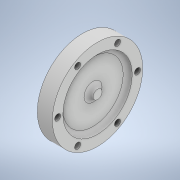
# Autodesk Inventor part: 711126 (Доделать)
Saved by Autodesk Inventor 2022 (Build 260153000, 153)
## iProperties
Created: 2021-10-21
Part Number: 711126 (Доделать)
Material: Типовые
Document SubType Name: Modeling
Designer: RaNSiD
Density: 1 g/cm^3
Appearance: По умолчанию
Author: RaNSiD
Autodesk Inventor part; units mm, degrees
ref_plane "YZ Plane" through (0, 0, 0) normal (1, 0, 0) x (0, 1, 0)
ref_plane "XZ Plane" through (0, 0, 0) normal (0, 1, 0) x (-1, 0, 0)
ref_plane "XY Plane" through (0, 0, 0) normal (0, 0, 1) x (1, 0, 0)
sketch "Эскиз1" plane through (0, 0, 0) normal (0, 0, 1) x (1, 0, 0)
  line L0 (0, 0) -> (10, 0)
  line L1 (10, 0) -> (10, 30)
  line L2 (10, 30) -> (0, 30)
  line L3 (0, 30) -> (0, 0)
  dimension "d0" = 10
  dimension "d1" = 30
  constraints: 8 end point, 2 parallel, 1 horizontal, 1 perpendicular
  measures "d0" distance of L2.end L1.end
  measures "d1" distance of L1.end L0.end
revolve "Вращение1" add sketch "Эскиз1" angle 360 about axis through (0, 0, 0) along (1, 0, 0)
sketch "Эскиз2" plane through (0, 0, 0) normal (0, 0, 1) x (1, 0, 0)
  line L0 (0, 0) -> (10, 0)
  line L1 (10, -30) -> (10, 30) projected
  arc A0 (3, 20) -> (0, 23) centre (0, 20) ccw
  line L2 (3, 20) -> (0, 20) construction
  line L3 (0, 23) -> (0, 20) construction
  line L4 (7, 20) -> (7, 10)
  arc A1 (7, 6) -> (10, 3) centre (10, 6) ccw
  line L5 (7, 6) -> (10, 6) construction
  line L6 (10, 3) -> (10, 6) construction
  arc A2 (10, 23) -> (7, 20) centre (10, 20) ccw
  line L7 (7, 20) -> (10, 20) construction
  line L8 (10, 23) -> (10, 20) construction
  line L9 (7, 10) -> (7, 6)
  line L10 (0, -30) -> (0, 30) projected
  line L11 (0, 0) -> (0, 23)
  line L12 (10, 3) -> (10, 23)
  line L13 (3, 20) -> (3, 0)
  point P0 (10, 3)
  point P1 (10, 23)
  dimension "d4" = 3
  dimension "d5" = 90
  dimension "d6" = 3
  dimension "d7" = 90
  dimension "d8" = 3
  dimension "d9" = 90
  dimension "d10" = 3
  dimension "d12" = 20
  dimension "d14" = 20
  constraints: 24 end point, 6 point on circle, 5 tangent, 3 centre point, 2 vertical, 2 vertical alignment, 1 horizontal alignment, 1 midpoint, 1 perpendicular, 1 point on line
  measures "d4" radius of A0
  measures "d5" angle of L2 L3
  measures "d6" radius of A1
  measures "d7" angle of L5 L6
  measures "d8" radius of A2
  measures "d9" angle of L8 L7
  measures "d10" distance of L0.end L6.start
  measures "d12" diameter of L4.end L0
  measures "d14" distance of L2.start L13.end
revolve "Вращение2" cut sketch "Эскиз2" angle 360 about axis through (0, 0, 0) along (-1, 0, 0) contours A1 L9 L4 A2 L1
sketch "Эскиз3" plane through (10, 0, 0) normal (1, 0, 0) x (0, 0, -1)
  point P0 (0, 0)
  point P1 (26.5, 0)
  point P2 (13.25, 22.9497)
  point P3 (-13.25, 22.9497)
  point P4 (-26.5, 0)
  point P5 (-13.25, -22.9497)
  point P6 (13.25, -22.9497)
  dimension "d15" = 26.5
  dimension "d18" = 360
  constraints: 7 other
  measures "d15" distance of point (0, 0) point (26.5, 0)
hole "Отверстие1" at (10, 0, -26.5) at (10, 22.9497, -13.25) at (10, 22.9497, 13.25) at (10, 0, 26.5) at (10, -22.9497, 13.25) at (10, -22.9497, -13.25) direction (-1, 0, 0) diameter 4 depth 16
